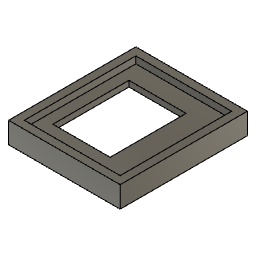
weather_station_light_sensor_top v12 (Autodesk Fusion 360 design; units mm, degrees)
Autodesk Fusion 360 part; units mm, degrees
sketch "Sketch1" plane through (0, 0, 0) normal (0, 0, 1) x (1, 0, 0)
  line L0 (0, 0) -> (16.5, 0)
  line L1 (16.5, 0) -> (16.5, 19.43)
  line L2 (16.5, 19.43) -> (0, 19.43)
  line L3 (0, 19.43) -> (0, 0)
  line L4 (0, 19.43) -> (1.2, 19.43)
  line L5 (1.2, 0) -> (0, 0)
  line L6 (0, 0) -> (0, 19.43)
  line L7 (16.5, 19.43) -> (13.5, 19.43)
  line L8 (13.5, 19.43) -> (13.5, 0)
  line L9 (13.5, 0) -> (16.5, 0)
  line L10 (16.5, 0) -> (16.5, 19.43)
  line L11 (-4.4, -5.285) -> (21.9, -5.285)
  line L12 (21.9, -5.285) -> (21.9, 24.715)
  line L13 (21.9, 24.715) -> (-4.4, 24.715)
  line L14 (-4.4, 24.715) -> (-4.4, -5.285)
  line L15 (0, 0) -> (13.5, 0)
  line L16 (13.5, 0) -> (13.5, 0.75)
  line L17 (13.5, 0.75) -> (0, 0.75)
  line L18 (0, 0.75) -> (0, 0)
  line L19 (0, 19.43) -> (13.5, 19.43)
  line L20 (13.5, 19.43) -> (13.5, 18.68)
  line L21 (13.5, 18.68) -> (0, 18.68)
  line L22 (0, 18.68) -> (0, 19.43)
  line L23 (-2.55, -3.435) -> (20.05, -3.435)
  line L24 (20.05, -3.435) -> (20.05, 22.865)
  line L25 (20.05, 22.865) -> (-2.55, 22.865)
  line L26 (-2.55, 22.865) -> (-2.55, -3.435)
  dimension "d1" = 16.5
  dimension "d2" = 19.43
  dimension "d4" = 3
  dimension "d9" = 4.4
  dimension "d49" = 0.75
  dimension "d50" = 0.75
  dimension "d53" = 30
  dimension "d54" = 5.285
  dimension "d55" = 1.85
  dimension "d56" = 1.85
  dimension "d57" = 1.85
  dimension "d58" = 1.85
  dimension "d71" = 5.4
  dimension "d72" = 25.3
  constraint horizontal L0
  constraint vertical L1
  constraint horizontal L2
  constraint vertical L3
  constraint coincident L0.start L3.end
  constraint horizontal L4
  constraint horizontal L5
  constraint vertical L6
  constraint horizontal L7
  constraint vertical L8
  constraint horizontal L9
  constraint vertical L10
  constraint coincident L0 L8.end
  constraint horizontal L11
  constraint vertical L12
  constraint horizontal L13
  constraint vertical L14
  constraint horizontal L15
  constraint vertical L16
  constraint horizontal L17
  constraint vertical L18
  constraint horizontal L19
  constraint vertical L20
  constraint horizontal L21
  constraint vertical L22
  constraint coincident L8 L20.end
  constraint horizontal L23
  constraint vertical L24
  constraint horizontal L25
  constraint vertical L26
  constraint coincident L8 L16.end
  measures "d1" distance of L0.start L0.end
  measures "d2" distance of L0.start L2.end
  measures "d4" distance of L1.end L7.end
  measures "d9" distance of L6 L14
  measures "d49" distance of L0.start L17.end
  measures "d50" distance of L19 L21
  measures "d53" distance of L11.start L13.end
  measures "d54" distance of L0 L11
  measures "d55" distance of L12 L24
  measures "d56" distance of L11 L23
  measures "d57" distance of L14 L26
  measures "d58" distance of L13 L25
  measures "d71" distance of L1 L12
extrude "Extrude14" add sketch "Sketch1" along normal blind 1.62 contours L11 L12 L13 L14
extrude "Extrude15" add sketch "Sketch1" against normal blind 3.38 contours L11 L12 L13 L14
extrude "Extrude16" add sketch "Sketch1" against normal blind 1.38 contours L0 L3 L5 L6 L8 L15 L16 L17 L18 | L0 L1 L2 L7 L8 L9 L10 L16 L20 | L2 L3 L4 L6 L8 L19 L20 L21 L22 | L23 L24 L25 L26
equation "d32 = ( 16.50 mm - d27 ) / 2"
equation "d49 = d50"
equation "d54 = ( d53 - d2 ) / 2"
equation "d56 = d55"
equation "d57 = d55"
equation "d58 = d55"
equation "d80 = -1.38 mm"
equation "d24 = 3.2 mm"
equation "d25 = d24"
equation "d26 = 10 mm"
equation "d27 = ( 30 mm - d26 ) / 2"
equation "d29 = ( 6.4 / sin(45 °) ) * 1 mm"
equation "d81 = d80 / 2"
